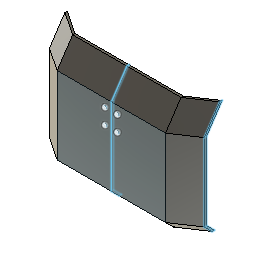
shovel (Autodesk Fusion 360 design; units mm, degrees)
Autodesk Fusion 360 part; units mm, degrees
sketch "Skizze1" plane through (0, 0, 0) normal (1, 0, 0) x (0, 1, 0)
  line L0 (50, 0) -> (40, 10)
  line L1 (40, 10) -> (40, 110)
  line L2 (40, 110) -> (60, 140)
  line L3 (47, 0) -> (37, 10)
  line L4 (37, 10) -> (37, 110)
  line L5 (37, 110) -> (57, 140)
  line L6 (57, 140) -> (60, 140)
  line L7 (47, 0) -> (50, 0)
  constraint vertical L1
  constraint parallel L0 L3
  constraint vertical L4
  constraint horizontal L6
  constraint parallel L6 L7
extrude "Extrusion1" add sketch "Skizze1" along normal mid plane 140 makes body 1
sketch "Skizze2" plane through (0, 0, 0) normal (1, 0, 0) x (0, 1, 0)
  line L0 (67, 0, 100) -> (70, 0, 100)
  line L1 (70, 0, 100) -> (60, 10, 100)
  line L2 (60, 10, 100) -> (60, 110, 100)
  line L3 (77, 140, 100) -> (80, 140, 100)
  line L4 (60, 110, 100) -> (80, 140, 100)
  line L5 (67, 0, 100) -> (57, 10, 100)
  line L6 (57, 110, 100) -> (77, 140, 100)
  line L7 (57, 10, 100) -> (57, 110, 100)
loft "Erhebung1" add profiles "Skizze2" section 1 face at (70, 38, 76.6667) section 2 contours L0 L1 L2 L3 L4 L5 L6 L7 in plane through (100, 0, 0) normal (1, 0, 0) separate body on bodies 1 makes body 2
mirror "Spiegeln1" about plane through (0, 0, 0) normal (1, 0, 0) of bodies 2 makes body 3
sketch "Skizze3" plane through (0, 37, 0) normal (0, -1, 0) x (1, 0, 0)
  line L0 (-70, 10) -> (70, 10)
  line L1 (70, 10) -> (70, 110)
  line L2 (70, 110) -> (-70, 110)
  line L3 (-70, 110) -> (-70, 10)
  circle A0 centre (-8, 100) radius 1.75
  circle A1 centre (8, 100) radius 1.75
  circle A2 centre (-8, 80) radius 1.75
  circle A3 centre (8, 80) radius 1.75
  dimension "d5" = 3.5
  dimension "d6" = 3.5
  dimension "d7" = 3.5
  dimension "d8" = 3.5
  measures "d5" diameter of A0
  measures "d6" diameter of A1
  measures "d7" diameter of A2
  measures "d8" diameter of A3
extrude "Extrusion2" cut sketch "Skizze3" against normal blind 3 contours A0 | A1 | A2 | A3 bodies 1
